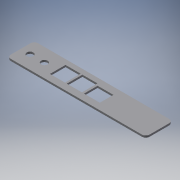
# Autodesk Inventor part: case-back
Saved by Autodesk Inventor 2017 (Build 210142000, 142)
## iProperties
Created: 2020-10-01
Part Number: case-back
Material: Generic
Document SubType Name: Modeling
Designer: jferner
Density: 1 g/cm^3
Appearance: Default
Author: jferner
Autodesk Inventor part; units mm, degrees
ref_plane "YZ Plane" through (0, 0, 0) normal (1, 0, 0) x (0, 1, 0)
ref_plane "XZ Plane" through (0, 0, 0) normal (0, 1, 0) x (-1, 0, 0)
ref_plane "XY Plane" through (0, 0, 0) normal (0, 0, 1) x (1, 0, 0)
sketch "Sketch1" plane through (0, 0, 0) normal (0, 0, 1) x (1, 0, 0)
  line L0 (-4, 0) -> (-144, 0)
  line L1 (-148, 4) -> (-148, 25)
  line L2 (-144, 29) -> (-4, 29)
  line L3 (0, 25) -> (0, 4)
  arc A0 (0, 25) -> (-4, 29) centre (-4, 25) ccw
  arc A1 (-144, 29) -> (-148, 25) centre (-144, 25) ccw
  arc A2 (-148, 4) -> (-144, 0) centre (-144, 4) ccw
  arc A3 (-4, 0) -> (0, 4) centre (-4, 4) ccw
  point P0 (0, 0)
  point P1 (-148, 0)
  point P2 (0, 29)
  dimension "d0" = 148
  dimension "d1" = 29
  dimension "d2" = 4
  constraints: 8 end point, 8 point on circle, 8 tangent, 6 point on line, 4 centre point, 3 equal radius, 2 parallel, 1 horizontal, 1 perpendicular
  measures "d0" distance of point (0, 0) point (-148, 0)
  measures "d1" distance of point (0, 29) point (0, 0)
  measures "d2" radius of A0
extrude "Extrusion1" add sketch "Sketch1" along normal blind 2
sketch "Sketch2" plane through (0, 0, 0) normal (0, 0, -1) x (-1, 0, 0)
  line L0 (55.9784, 21.4874) -> (72.8534, 21.4874)
  line L1 (72.8534, 21.4874) -> (72.8534, 7)
  line L2 (72.8534, 7) -> (55.9784, 7)
  line L3 (55.9784, 7) -> (55.9784, 21.4874)
  line L4 (144, 0) -> (4, 0) projected
  line L5 (0, 4) -> (0, 25) projected
  line L6 (75.1046, 23.6) -> (91.2046, 23.6)
  line L7 (91.2046, 23.6) -> (91.2046, 7)
  line L8 (91.2046, 7) -> (75.1046, 7)
  line L9 (75.1046, 7) -> (75.1046, 23.6)
  line L10 (93.1046, 23.6) -> (109.2046, 23.6)
  line L11 (109.2046, 23.6) -> (109.2046, 7)
  line L12 (109.2046, 7) -> (93.1046, 7)
  line L13 (93.1046, 7) -> (93.1046, 23.6)
  circle A0 centre (122.7, 14.5) radius 3.5
  circle A1 centre (138, 14.5) radius 3.5
  line L14 (148, 25) -> (148, 4) projected
  point P0 (0, 0)
  dimension "d7" = 16.875
  dimension "d8" = 14.4874
  dimension "d9" = 7
  dimension "d11" = 2.2512
  dimension "d12" = 1.9
  dimension "d13" = 16.1
  dimension "d14" = 16.1
  dimension "d15" = 16.6
  dimension "d16" = 7
  dimension "d17" = 7
  dimension "d18" = 7.5
  dimension "d19" = 13.4954
  dimension "d20" = 15.3
  dimension "d21" = 10
  constraints: 24 end point, 6 parallel, 3 horizontal, 3 perpendicular, 2 centre point, 2 collinear, 1 horizontal alignment, 1 point on line
  measures "d7" distance of L1.end L2.end
  measures "d8" distance of L2.end L0.start
  measures "d9" distance between parallel lines of L4 L2
  measures "d11" distance between parallel lines of L9 L1
  measures "d12" distance between parallel lines of L13 L7
  measures "d13" distance between parallel lines of L7 L9
  measures "d14" distance between parallel lines of L11 L13
  measures "d15" distance between parallel lines of L10 L12
  measures "d16" diameter of A0
  measures "d17" diameter of A1
  measures "d18" distance from line of L12 A0.centre
  measures "d19" distance from line of A0.centre L11
  measures "d20" distance of A1.centre A0.centre
  measures "d21" distance from line of L14 A1.centre
extrude "Extrusion2" cut sketch "Sketch2" against normal through all
equation "\"d0\" = caseBottomWidth - thickness"
equation "\"d1\" = -thickness + 2 * caseBottomHeight - lipHeight"
equation "\"d2\" = filletMid"
equation "\"d3\" = thickness"
equation "\"d14\" = d13"
equation "\"d5\" = thickness"
equation "\"filletMid\" = 4"
equation "\"thickness\" = 2"
equation "\"caseBottomWidth\" = 150"
equation "\"caseBottomHeight\" = 16"
equation "\"lipHeight\" = 1"
body "Solid1"
